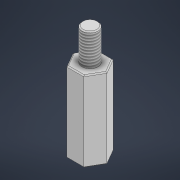
# Autodesk Inventor part: Spacer_M3_Hex-L15-Bolt
Saved by Autodesk Inventor 2022.4 (Build 264492010, 492A)
## iProperties
Created: 2023-06-19
Part Number: Spacer_M3_Hex-L15-Bolt
Material: 一般
Document SubType Name: Modeling
Designer: 22-ayato
Density: 1 g/cm^3
Appearance: 既定
Author: 22-ayato
Autodesk Inventor part; units mm, degrees
ref_plane "YZ Plane" through (0, 0, 0) normal (1, 0, 0) x (0, 1, 0)
ref_plane "XZ Plane" through (0, 0, 0) normal (0, 1, 0) x (-1, 0, 0)
ref_plane "XY Plane" through (0, 0, 0) normal (0, 0, 1) x (1, 0, 0)
sketch "スケッチ1" plane through (0, 0, 0) normal (0, 1, 0) x (-1, 0, 0)
  line L0 (1.5877, 2.75) -> (3.1754, 0)
  line L1 (3.1754, 0) -> (1.5877, -2.75)
  line L2 (1.5877, -2.75) -> (-1.5877, -2.75)
  line L3 (-1.5877, -2.75) -> (-3.1754, 0)
  line L4 (-3.1754, 0) -> (-1.5877, 2.75)
  line L5 (-1.5877, 2.75) -> (1.5877, 2.75)
  point P0 (0, 0)
  point P1 (0, 0)
  dimension "d1" = 5.5
  constraints: 12 end point, 1 coincident, 1 horizontal alignment, 13 other
  measures "d1" distance between parallel lines of L2 L5
extrude "押し出し1" add sketch "スケッチ1" along normal mid plane 15
sketch "スケッチ2" plane through (0, -7.5, 0) normal (0, -1, 0) x (1, 0, 0)
  point P0 (0, 0)
  point P1 (0, 0)
  constraints: 1 coincident
hole "穴1" at (0, -7.5, 0) direction (0, 1, 0) diameter 2.459 depth 12 tip angle 118 thread size "M3x0.5" class "6H" standard "ISO Metric profile"
sketch "スケッチ3" plane through (0, 7.5, 0) normal (0, 1, 0) x (1, 0, 0)
  circle A0 centre (0, 0) radius 1.5
  dimension "d11" = 3
  constraints: 1 centre point, 1 coincident
  measures "d11" diameter of A0
extrude "押し出し2" add sketch "スケッチ3" along normal blind 6
thread "ねじ1" size "M3x0.5" class "6g" standard "ANSI Metric M Profile" full length
chamfer "面取り1" distance 0.2 angle 45 1 edges at (-1.5, 13.5, 0)
chamfer "面取り2" distance 0.2 angle 45 13 edges at (2.3816, 7.5, 1.375) (2.3816, 7.5, -1.375) (0, 7.5, -2.75) (-2.3816, 7.5, -1.375) (-2.3816, 7.5, 1.375) (0, 7.5, 2.75) (0, -7.5, 2.75) (2.3816, -7.5, 1.375) (2.3816, -7.5, -1.375) (0, -7.5, -2.75) (-2.3816, -7.5, -1.375) (-2.3816, -7.5, 1.375) (0, -7.5, 1.2295)
